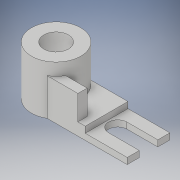
# Autodesk Inventor part: Distance from Face Complete
Saved by Autodesk Inventor 2018 (Build 220105000, 105)
## iProperties
Created: 2017-03-08
Part Number: Distance from Face Complete
Material: Generic
Document SubType Name: Modeling
Designer: John Helfen
Density: 1 g/cm^3
Appearance: Default
Author: John Helfen
Autodesk Inventor part; units mm, degrees
ref_plane "YZ Plane" through (0, 0, 0) normal (1, 0, 0) x (0, 1, 0)
ref_plane "XZ Plane" through (0, 0, 0) normal (0, 1, 0) x (-1, 0, 0)
ref_plane "XY Plane" through (0, 0, 0) normal (0, 0, 1) x (1, 0, 0)
sketch "Sketch1" plane through (0, 0, 0) normal (0, 1, 0) x (-1, 0, 0)
  circle A0 centre (0, 0) radius 12.7
  circle A1 centre (0, 0) radius 25.4
  line L0 (-12.7, -21.997) -> (-95.25, -21.997)
  line L1 (-95.25, 21.997) -> (-12.7, 21.997)
  arc A2 (-63.5, -9.525) -> (-63.5, 9.525) centre (-63.5, 0) ccw
  line L2 (-63.5, 9.525) -> (-95.25, 9.525)
  line L3 (-78.5703, 0) -> (-63.5, 0) construction
  line L4 (-63.5, -9.525) -> (-95.25, -9.525)
  line L5 (-95.25, -21.997) -> (-95.25, -9.525)
  line L6 (-95.25, 9.525) -> (-95.25, 21.997)
  line L7 (-44.45, 21.997) -> (-44.45, 12.472)
  line L8 (-44.45, 12.472) -> (-22.1271, 12.472)
  line L9 (-52.07, 21.997) -> (-52.07, -21.997)
  dimension "d0" = 25.4
  dimension "d3" = 19.05
  dimension "d4" = 31.75
  dimension "d5" = 12.7
  dimension "d6" = 44.45
  dimension "d7" = 9.525
  dimension "d8" = 7.62
  dimension "d9" = 82.55
  dimension "d10" = 12.7
  constraints: 20 end point, 6 perpendicular, 5 point on circle, 3 centre point, 3 horizontal, 3 point on line, 2 coincident, 2 equal length, 2 tangent, 1 collinear, 1 parallel, 1 vertical
  measures "d0" diameter of A0
  measures "d3" diameter of A2
  measures "d4" distance of L2.start L2.end
  measures "d5" horizontal distance of point (0, 0) L1.end
  measures "d6" distance from line of point (0, 0) L7
  measures "d7" distance between parallel lines of L1 L8
  measures "d8" distance between parallel lines of L7 L9
  measures "d9" distance of L0.start L0.end
  measures "d10" radial gap between concentric circles of A0 A1
extrude "Extrusion3" add sketch "Sketch1" along normal blind 50.8 contours A1
extrude "Extrusion4" add sketch "Sketch1" along normal blind 6.35 contours A1 L8 L7 L1 | L0 L9 L1 L7 L8 A1 | L0 L5 L4 A2 L2 L6 L1 L9
extrude "Extrusion5" add sketch "Sketch1" along normal blind 6.35 from surface at 6.35 contours A1 L8 L7 L1 | L0 L9 L1 L7 L8 A1
extrude "Extrusion6" add sketch "Sketch1" along normal blind 25.4 from surface at 12.7 contours A1 L8 L7 L1
body "Solid2"
